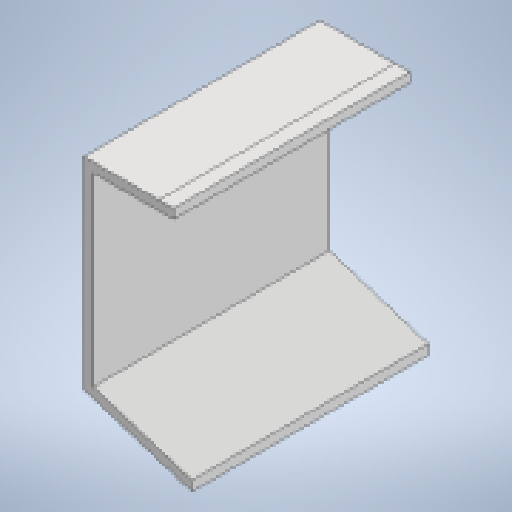
# Autodesk Inventor part: nozzz
Saved by Autodesk Inventor 2023 (Build 270158000, 158)
## iProperties
Created: 2023-07-30
Part Number: nozzz
Material: Stal, węglowa
Document SubType Name: Modeling
Designer: Kamil
Density: 7.85 g/cm^3
Appearance: Częściowo polerowany
Author: Kamil
Autodesk Inventor part; units mm, degrees
ref_plane "YZ Plane" through (0, 0, 0) normal (1, 0, 0) x (0, 1, 0)
ref_plane "XZ Plane" through (0, 0, 0) normal (0, 1, 0) x (-1, 0, 0)
ref_plane "XY Plane" through (0, 0, 0) normal (0, 0, 1) x (1, 0, 0)
sketch "Szkic1" plane through (0, 0, 0) normal (0, 0, 1) x (1, 0, 0)
  line L0 (0, -50) -> (2, -50) projected
  circle A0 centre (-3.1, -7) radius 7 projected
  line L1 (3.9, -50) -> (3.9, 0)
  line L2 (3.9, -50) -> (-19.6026, -42.4936)
  line L3 (2, -14) -> (2, -47.2936) projected
  line L4 (0, -14) -> (0, -46.6549) projected
  line L5 (3.9, -47.9005) -> (-27.3591, -37.9167)
  line L6 (-14, -40.7018) -> (-14, -39.1018) projected
  line L7 (-14, -40.7018) -> (-14, -42.2018)
  line L8 (-14, -39.1018) -> (-17, -39.1018)
  line L9 (-17, -41.2253) -> (-17, 0)
  line L10 (-17, 0) -> (-3.1, 0)
  line L11 (-19, -40.5865) -> (-19, 0.0005)
  line L12 (-19, 0.0005) -> (-3.1, 0.0005)
  line L13 (-3.1, -1.9995) -> (-19, -1.9995)
  line L14 (-19, -1.9995) -> (-19, 0.0005)
  line L15 (-19, -40.5865) -> (-19, -42.6861)
  line L16 (0, -14) -> (0, 0) projected
  line L17 (2, -14) -> (0, -14) projected
  line L18 (2, 0) -> (2, -14) projected
  line L19 (0, 0) -> (2, 0) projected
  line L20 (-3.1, 0) -> (0, 0)
  line L21 (-3.1, -1.9995) -> (0, -1.9995)
  line L22 (-19, 0.0005) -> (-17, 0.0005)
  line L23 (-17, 0.0005) -> (-17, -1.9995)
  line L24 (-17, -1.9995) -> (-19, -1.9995)
  line L25 (-19, -1.9995) -> (-19, 0.0005)
  dimension "d0" = 2
  dimension "d1" = 1.5
  dimension "d2" = 3
  dimension "d3" = 2
  dimension "d4" = 2
  constraints: 36 end point, 7 point on line, 6 parallel, 6 vertical, 4 horizontal, 3 perpendicular, 2 point on circle, 2 other
  measures "d0" distance between parallel lines of L5 L2
  measures "d1" distance of L6.start L7.end
  measures "d2" distance of L6.end L8.end
  measures "d3" distance between parallel lines of L9 L11
  measures "d4" distance of L12.end L13.start
extrude "Wyciągnięcie proste1" add sketch "Szkic1" against normal blind 50 contours L1 L2 L15 L5 | L16 L21 L13 A0 | A0 L20 L16 | A0 L13 L9 L10 | L9 L13 L11 L12 | L9 L5 L11 L13 picked at (-1.3641, -1.4413)
